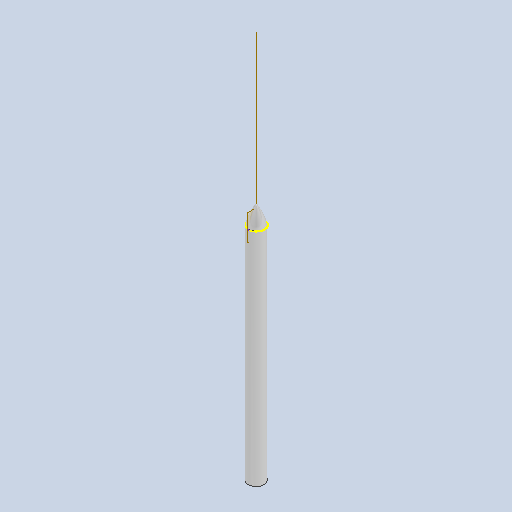
# Autodesk Inventor part: foot_claw_2.5
Saved by Autodesk Inventor 2023.1 (Build 271208000, 208)
## iProperties
Created: 2021-03-24
Part Number: foot_claw_2.5
Material: Generic
Document SubType Name: Modeling
Designer: JojoS
Density: 1 g/cm^3
Appearance: Aluminum - Polished
Author: JojoS
Autodesk Inventor part; units mm, degrees
ref_plane "YZ Plane" through (0, 0, 0) normal (1, 0, 0) x (0, 1, 0)
ref_plane "XZ Plane" through (0, 0, 0) normal (0, 1, 0) x (-1, 0, 0)
ref_plane "XY Plane" through (0, 0, 0) normal (0, 0, 1) x (1, 0, 0)
sketch "Sketch1" plane through (0, 0, 0) normal (0, 1, 0) x (-1, 0, 0)
  circle A0 centre (0, 0) radius 0.5
  dimension "d0" = 1
  constraints: 1 centre point, 1 coincident
  measures "d0" diameter of A0
extrude "Extrusion1" add sketch "Sketch1" along normal blind 14
sketch "Sketch2" plane through (0, 14, 0) normal (0, 1, 0) x (1, 0, 0)
  circle A0 centre (0, 0) radius 0.5 projected
  line L0 (0, -0.5) -> (0, 0.5)
  constraints: 2 end point, 2 point on circle, 1 vertical
ref_plane "Work Plane2" through (0, 14, 0.5) normal (1, 0, 0) x (0, 0, -1)
sketch "Sketch3" plane through (0, 14, 0.5) normal (1, 0, 0) x (0, 0, -1)
  line L0 (1, 0) -> (0, 0) projected
  line L1 (0.5, 0) -> (0.5, 1.2)
  arc A0 (1, 0) -> (0.5, 1.2) centre (-2.6017, -0.7966) ccw
  line L2 (0.5, -24.2444) -> (0.5, 5.4666) projected
  point P0 (0.5, -14)
  dimension "d4" = 1.2
  constraints: 2 end point, 2 point on circle, 1 centre point, 1 midpoint, 1 vertical
  measures "d4" distance of L1.start L1.end
revolve "Revolution1" add sketch "Sketch3" angle 360 about axis through (0, 14, 0) along (0, 1, 0)
body "Solid1"
